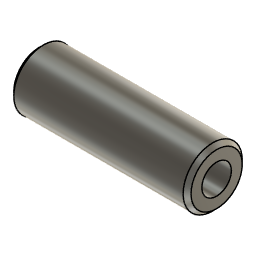
Single cylider engin (Autodesk Fusion 360 archive; units mm, degrees)
design "Piston+Pin_"
Autodesk Fusion 360 part; units mm, degrees
note: some values were not read from the file. Chosen so that the rebuilt part matches the saved one: a direction. Set by a fixed rule: which sketch regions a step uses.
sketch "Sketch1" plane through (0, 0, 0) normal (1, 0, 0) x (0, 1, 0)
  circle A0 centre (0, 0) radius 15
  circle A1 centre (0, 0) radius 7.5
  dimension "d1" = 30
  dimension "d2" = 15
  constraint coincident A0.centre A1.centre
  constraint concentric A0 A1
  measures "d1" diameter of A0
  measures "d2" diameter of A1
extrude "Extrude1" add sketch "Sketch1" along normal mid plane 90
chamfer "Chamfer1" distance 2 angle 45 2 edges at (45, -13.9849, -5.4242) (-45, -13.9849, 5.4242)

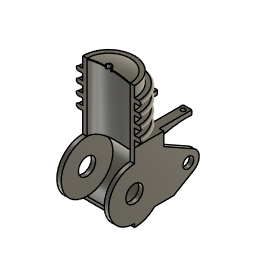
design "Crank+Case_"
Autodesk Fusion 360 part; units mm, degrees
sketch "Sketch1" plane through (0, 0, 0) normal (1, 0, 0) x (0, 1, 0)
  line L0 (0, 0) -> (0, 160)
  line L1 (0, 160) -> (68, 160)
  line L2 (68, 160) -> (68, 68)
  arc A0 (0, 0) -> (68, 68) centre (0, 68) ccw
  dimension "d1" = 160
  dimension "d2" = 68
  dimension "d3" = 68
  constraint coincident L0.start A0.start
  constraint vertical L0
  constraint perpendicular L0 L1
  constraint perpendicular L1 L2
  constraint tangent L2 A0
  measures "d1" distance of L0.start L0.end
  measures "d2" distance of L0.end L1.end
  measures "d3" radius of A0
extrude "Extrude1" add sketch "Sketch1" along normal mid plane 120
sketch "Sketch2" plane through (0, 0, 0) normal (0, -1, 0) x (1, 0, 0)
  line L0 (-60, 0) -> (60, 0)
  line L1 (60, 0) -> (60, 160)
  line L2 (60, 160) -> (-60, 160)
  line L3 (-60, 160) -> (-60, 0)
  line L4 (60, 185) -> (60, 200)
  line L5 (60, 175) -> (70, 175)
  line L6 (60, 225) -> (70, 225)
  line L7 (70, 185) -> (60, 185)
  line L8 (70, 235) -> (60, 235)
  line L9 (60, 260) -> (60, 285)
  line L10 (5, 295) -> (5, 286)
  line L11 (7, 291) -> (7, 295)
  line L12 (5, 286) -> (7, 286)
  arc A0 (70, 200) -> (70, 210) centre (70, 205) ccw
  line L13 (7, 295) -> (5, 295)
  line L14 (70, 260) -> (60, 260)
  arc A1 (70, 175) -> (70, 185) centre (70, 180) ccw
  line L15 (7, 286) -> (7, 289)
  line L16 (60, 285) -> (50, 285)
  line L17 (60, 250) -> (70, 250)
  line L18 (60, 235) -> (60, 250)
  arc A2 (70, 250) -> (70, 260) centre (70, 255) ccw
  arc A3 (70, 225) -> (70, 235) centre (70, 230) ccw
  line L19 (50, 160) -> (50, 282.9194)
  line L20 (60, 210) -> (60, 225)
  line L21 (70, 210) -> (60, 210)
  line L22 (0, 0) -> (0, 288.3131) construction
  line L23 (60, 200) -> (70, 200)
  line L24 (60, 160) -> (60, 175)
  line L25 (50, 160) -> (60, 160)
  arc A4 (50, 285) -> (7, 291) centre (7.0116, 134) ccw
  arc A5 (50, 282.9194) -> (7, 289) centre (7.0116, 134) ccw
  dimension "d12" = 25
  dimension "d13" = 0
  dimension "d14" = 5
  dimension "d15" = 20
  dimension "d16" = 125
  dimension "d17" = 10
  dimension "d19" = 100
  dimension "d20" = 10
  dimension "d21" = 14
  dimension "d22" = 9
  dimension "d23" = 3
  dimension "d29" = 135
  dimension "d30" = 10
  dimension "d31" = 157
  dimension "d32" = 155
  constraint coincident L22.start origin
  constraint perpendicular L5 L24
  constraint tangent L5 A1
  constraint coincident L4.start L24
  constraint tangent L7 A1
  constraint perpendicular L7 L24
  constraint collinear L4 L24
  constraint collinear L4 L20
  constraint collinear L18 L20
  constraint collinear L9 L18
  constraint perpendicular L9 L16
  constraint vertical L10
  constraint perpendicular L10 L12
  constraint perpendicular L12 L15
  constraint horizontal L13
  constraint coincident L11.start L15
  constraint collinear L11 L15
  constraint coincident L2 L1.end
  constraint coincident L1 L2.start
  constraint coincident L2 L19.start
  constraint concentric A4 A5
  measures "d14" radius of A1
  measures "d15" vertical distance of A1.centre L1.end
  measures "d16" vertical distance of L1.end L9.end
  measures "d17" horizontal distance of A1.centre L1.end
  measures "d22" vertical distance of L10.start L10.end
  measures "d23" distance of L15.end L12
  measures "d29" distance of L13 L25
  measures "d30" distance of L9.end L16.end
  measures "d31" radius of A4
  measures "d32" radius of A5
revolve "Revolve1" add sketch "Sketch2" angle 180 about axis through (0, 0, 0) along (0, 0, 1) contours L2 L4 L5 L6 L7 L8 L9 L10 L11 L12 A0 L13 L14 A1 L15 L16 L17 L18 A2 A3 L19 L20 L21 L23 L24 L25 A4 A5
sketch "Sketch3" plane through (60, 0, 0) normal (1, 0, 0) x (0, 1, 0)
  line L0 (0, 160) -> (0, 0)
  arc A0 (0, 0) -> (68, 68) centre (0, 68) ccw
  line L1 (68, 68) -> (68, 160)
  line L2 (68, 160) -> (0, 160)
  circle A1 centre (0, 68) radius 60
  dimension "d34" = 120
  constraint concentric A0 A1
  measures "d34" diameter of A1
extrude "Extrude2" cut sketch "Sketch3" against normal through all contours L0 A1 | L0 A1
sketch "Sketch4" plane through (0, 0, 160) normal (0, 0, 1) x (-1, 0, 0)
  arc A0 (-50, 0) -> (50, 0) centre (0, 0) ccw
  line L0 (50, 0) -> (-50, 0)
  circle A1 centre (0, 0) radius 50
  constraint concentric A0 A1
  constraint equal A0 A1
extrude "Extrude3" cut sketch "Sketch4" along normal up to surface end surface at (-20, 5.9741, 8.2982)
sketch "Sketch6" plane through (60, 0, 0) normal (1, 0, 0) x (0, 1, 0)
  arc A0 (0, 8) -> (0, 128) centre (0, 68) ccw
  line L0 (0, 8) -> (0, 0)
  arc A1 (0, 0) -> (68, 68) centre (0, 68) ccw
  line L1 (68, 68) -> (68, 160)
  line L2 (68, 160) -> (0, 160)
  line L3 (0, 160) -> (0, 128)
  circle A2 centre (0, 68) radius 60
  circle A3 centre (0, 68) radius 20
  dimension "d38" = 40
  constraint concentric A0 A2
  constraint equal A0 A2
  constraint concentric A2 A3
  measures "d38" diameter of A3
extrude "Extrude4" add sketch "Sketch6" against normal blind 10 contours A0 A2
mirror "Mirror1" about plane through (0, 0, 0) normal (1, 0, 0) of "Extrude4"
sketch "Sketch7" plane through (60, 0, 0) normal (1, 0, 0) x (0, 1, 0)
  circle A0 centre (0, 68) radius 20
  line L0 (0, 8) -> (0, 0)
  arc A1 (0, 0) -> (68, 68) centre (0, 68) ccw
  line L1 (68, 68) -> (68, 160)
  line L2 (68, 160) -> (0, 160)
  line L3 (0, 160) -> (0, 128)
  arc A2 (0, 128) -> (0, 8) centre (0, 68) ccw
  line L4 (90.9301, 18.7906) -> (137.7314, 46.4846)
  arc A3 (137.7314, 46.4846) -> (137.2671, 89.7834) centre (125, 68) ccw
  line L5 (137.2671, 89.7834) -> (68, 128.7906)
  line L6 (46.9301, 18.7906) -> (90.9301, 18.7906)
  line L7 (0, 68) -> (188.2817, 68) construction
  circle A4 centre (125, 68) radius 12.5
  dimension "d42" = 44
  dimension "d43" = 25
  dimension "d45" = 60
  dimension "d46" = 110
  dimension "d47" = 125
  dimension "d51" = 25
  constraint tangent L4 A3
  constraint coincident L1 L5.end
  constraint tangent A3 L5
  constraint coincident A1 L6.start
  constraint horizontal L6
  constraint horizontal A0.centre A3.centre
  constraint coincident A0.centre A1.centre
  constraint horizontal L7
  constraint concentric A3 A4
  measures "d42" distance of L4.start L6.start
  measures "d43" radius of A3
  measures "d45" angle of L4 L5
  measures "d46" distance of L5.end L6
  measures "d47" horizontal distance of A0.centre A3.centre
  measures "d51" diameter of A4
extrude "Extrude5" add sketch "Sketch7" against normal blind 10 contours A1 L1 L4 A3 L5 L6
mirror "Mirror2" about plane through (0, 0, 0) normal (1, 0, 0) of "Extrude5"
ref_plane "WorkPlane1" through (50, 45.0767, 80) normal (1, 0, 0) x (0, 1, 0)
sketch "Sketch8" plane through (50, 45.0767, 80) normal (1, 0, 0) x (0, 1, 0)
  line L0 (22.9233, 80) -> (22.9233, 48.7906)
  line L1 (22.9233, 80) -> (97.9233, 80)
  line L2 (97.9233, 80) -> (97.9233, 70)
  arc A0 (97.9233, 70) -> (22.9233, 60) centre (86.3789, -129.6665) ccw
  line L3 (22.9233, 80) -> (22.9233, 60)
  point P0 (22.9233, 80)
  dimension "d53" = 75
  dimension "d54" = 10
  dimension "d55" = 200
  dimension "d56" = 20
  constraint coincident P0 L0.start
  constraint perpendicular L0 L1
  constraint perpendicular L1 L2
  constraint coincident L0 A0.end
  measures "d53" distance of P0 L1.end
  measures "d54" distance of L1.end L2.end
  measures "d55" radius of A0
  measures "d56" distance of A0.end P0
extrude "Extrude6" add sketch "Sketch8" against normal blind 20
sketch "Sketch9" plane through (0, 0, 160) normal (0, 0, 1) x (-1, 0, 0)
  arc A0 (-60, 0) -> (60, 0) centre (0, 0) ccw
  line L0 (-60, 0) -> (-60, -68)
  line L1 (-60, -68) -> (-50, -68)
  line L2 (-50, -68) -> (-50, -143)
  line L3 (-50, -143) -> (-30, -143)
  line L4 (-30, -143) -> (-30, -68)
  line L5 (-30, -68) -> (60, -68)
  line L6 (60, -68) -> (60, 0)
  circle A1 centre (-40, -133) radius 5
  dimension "d59" = 10
  dimension "d60" = 10
  dimension "d61" = 10
  measures "d59" diameter of A1
  measures "d60" distance of L3 A1.centre
  measures "d61" distance of L4 A1.centre
extrude "Extrude7" cut sketch "Sketch9" along normal up to surface contours A1 end surface at (36.6667, 134.5483, 150.3096)
mirror "Mirror3" about plane through (0, 0, 0) normal (1, 0, 0) of "Extrude6", "Extrude7"

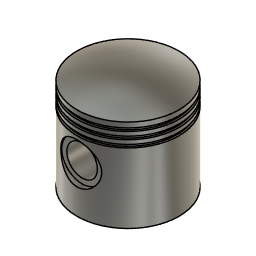
design "Piston_"
Autodesk Fusion 360 part; units mm, degrees
sketch "Sketch1" plane through (0, 0, 0) normal (0, 1, 0) x (1, 0, 0)
  line L0 (0, 0) -> (0, -80) construction
  line L1 (0, 0) -> (72.9805, 0) construction
  line L2 (50, 0) -> (50, -68.3994)
  line L3 (50, 0) -> (43, 0)
  line L4 (43, -20) -> (43, 0)
  line L5 (50, -68.3994) -> (48, -68.3994)
  line L6 (48, -68.3994) -> (48, -71.3994)
  line L7 (48, -71.3994) -> (50, -71.3994)
  line L8 (50, -71.3994) -> (50, -75.3994)
  line L9 (50, -75.3994) -> (48, -75.3994)
  line L10 (48, -75.3994) -> (48, -78.3994)
  line L11 (48, -78.3994) -> (50, -78.3994)
  line L12 (50, -78.3994) -> (50, -82.3994)
  line L13 (50, -82.3994) -> (48, -82.3994)
  line L14 (48, -82.3994) -> (48, -85.3994)
  line L15 (48, -85.3994) -> (50, -85.3994)
  line L16 (50, -85.3994) -> (50, -90.3994)
  arc A0 (0, -100) -> (50, -90.3994) centre (0, 35) ccw
  line L17 (37.5, -84) -> (37.5, -20)
  line L18 (43, -20) -> (37.5, -20)
  line L19 (0, -100) -> (0, -84)
  line L20 (0, -84) -> (37.5, -84)
  dimension "d1" = 100
  dimension "d2" = 86
  dimension "d3" = 20
  dimension "d4" = 3
  dimension "d5" = 2
  dimension "d6" = 4
  dimension "d7" = 5
  dimension "d8" = 135
  dimension "d9" = 75
  dimension "d10" = 100
  dimension "d11" = 16
  constraint coincident L0.start L1.start
  constraint vertical L0
  constraint perpendicular L0 L1
  constraint coincident L1 L2.start
  constraint perpendicular L1 L2
  constraint coincident L1 L3.end
  constraint perpendicular L1 L4
  constraint perpendicular L2 L5
  constraint perpendicular L5 L6
  constraint perpendicular L6 L7
  constraint perpendicular L5 L8
  constraint perpendicular L8 L9
  constraint perpendicular L9 L10
  constraint perpendicular L10 L11
  constraint perpendicular L11 L12
  constraint perpendicular L10 L13
  constraint perpendicular L13 L14
  constraint perpendicular L10 L15
  constraint perpendicular L15 L16
  constraint equal L6 L10
  constraint equal L10 L14
  constraint collinear L6 L10
  constraint collinear L10 L14
  constraint equal L8 L12
  constraint collinear L12 L16
  constraint collinear L8 L12
  constraint collinear L2 L8
  constraint coincident L0 A0.start
  constraint horizontal L18
  constraint parallel L0 L19
  constraint horizontal L20
  constraint vertical L0.start A0.centre
  measures "d3" distance of L3.end L4.start
  measures "d4" distance of L5.end L6.end
  measures "d5" distance of L2.end L5.end
  measures "d6" distance of L7.end L8.end
  measures "d7" distance of L15.end L16.end
  measures "d8" radius of A0
  measures "d10" distance of L1 A0.start
  measures "d11" distance of A0.start L19.end
revolve "Revolve1" add sketch "Sketch1" angle 360 about axis through (0, 0, 0) along (0, 0, 1)
sketch "Sketch2" plane through (0, 0, 0) normal (0, 1, 0) x (1, 0, 0)
  circle A0 centre (0, -45) radius 15
  dimension "d14" = 30
  dimension "d15" = 45
  constraint vertical origin A0.centre
  measures "d14" diameter of A0
  measures "d15" distance of origin A0.centre
extrude "Extrude1" cut sketch "Sketch2" along normal through all and the other way through all
ref_plane "WorkPlane1" through (0, -20, 0) normal (0, 1, 0) x (0, 0, 1)
sketch "Sketch4" plane through (0, -20, 0) normal (0, 1, 0) x (1, 0, 0)
  circle A0 centre (0, -45) radius 15
  circle A1 centre (0, -45) radius 20
  dimension "d25" = 30
  dimension "d26" = 45
  dimension "d27" = 40
  constraint vertical origin A0.centre
  constraint concentric A0 A1
  measures "d25" diameter of A0
  measures "d26" vertical distance of origin A0.centre
  measures "d27" diameter of A1
extrude "Extrude3" add sketch "Sketch4" along normal up to surface end surface at (19.5913, -31.9755, 49.6667)
mirror "Mirror2" about plane through (0, 0, 0) normal (0, 1, 0) of "Extrude3"
ref_plane "WorkPlane2" through (0, -50, 0) normal (0, 1, 0) x (0, 0, 1)
sketch "Sketch5" plane through (0, -50, 0) normal (0, 1, 0) x (1, 0, 0)
  circle A0 centre (0, -45) radius 20
  circle A1 centre (0, -45) radius 20
  dimension "d32" = 40
  constraint concentric A0 A1
  measures "d32" diameter of A0
extrude "Extrude4" cut sketch "Sketch5" along normal blind 5
mirror "Mirror3" about plane through (0, 0, 0) normal (0, 1, 0) of "Extrude4"
